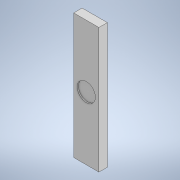
# Autodesk Inventor part: base
Saved by Autodesk Inventor 2021.2 (Build 252289000, 289)
## iProperties
Created: 2021-03-03
Part Number: base
Material: Generic
Document SubType Name: Modeling
Designer: zayda
Density: 1 g/cm^3
Appearance: Default
Author: zayda
Autodesk Inventor part; units mm, degrees
ref_plane "YZ Plane" through (0, 0, 0) normal (1, 0, 0) x (0, 1, 0)
ref_plane "XZ Plane" through (0, 0, 0) normal (0, 1, 0) x (-1, 0, 0)
ref_plane "XY Plane" through (0, 0, 0) normal (0, 0, 1) x (1, 0, 0)
ref_plane "Work Plane1" through (0, 0, 0) normal (0, 0, 1) x (1, 0, 0)
sketch "Sketch1" plane through (0, 0, 0) normal (0, 0, 1) x (1, 0, 0)
  line L0 (0, 0) -> (30.48, 0)
  line L1 (30.48, 0) -> (30.48, 152.4)
  line L2 (30.48, 152.4) -> (0, 152.4)
  line L3 (0, 152.4) -> (0, 0)
  dimension "d0" = 30.48
  dimension "d1" = 152.4
  constraints: 8 end point, 2 parallel, 1 horizontal, 1 perpendicular
  measures "d0" distance of L2.end L1.end
  measures "d1" distance of L1.end L0.end
extrude "Extrusion1" add sketch "Sketch1" along normal blind 10.16
sketch "Sketch2" plane through (0, 0, 10.16) normal (0, 0, 1) x (1, 0, 0)
  line L0 (0, 152.4) -> (0, 0) projected
  line L1 (0, 76.2) -> (30.48, 76.2)
  line L2 (30.48, 0) -> (30.48, 152.4) projected
  circle A0 centre (15.24, 76.2) radius 11.049
  dimension "d4" = 22.098
  constraints: 3 midpoint, 2 end point, 1 centre point
  measures "d4" diameter of A0
extrude "Extrusion2" cut sketch "Sketch2" against normal blind 1.5875
sketch "Sketch3" plane through (0, 152.4, 0) normal (0, 1, 0) x (1, 0, 0)
  line L0 (30.48, -10.16) -> (0, -10.16) projected
  line L1 (30.48, -10.16) -> (30.48, 0)
  line L2 (30.48, 0) -> (0, 0) projected
  line L3 (30.48, 0) -> (0, 0)
  line L4 (0, 0) -> (0, -10.16) projected
  line L5 (0, 0) -> (0, -10.16)
  line L6 (0, -10.16) -> (30.48, -10.16)
  constraints: 8 end point, 3 perpendicular, 1 vertical
extrude "Extrusion3" cut sketch "Sketch3" against normal blind 1.016
body "Solid1"
